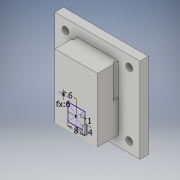
# Autodesk Inventor part: ChipMount
Saved by Autodesk Inventor 2019 (Build 230136000, 136)
## iProperties
Created: 2019-05-13
Part Number: ChipMount
Material: Generic
Document SubType Name: Modeling
Designer: aorfi
Density: 1 g/cm^3
Appearance: Default
Author: aorfi
Autodesk Inventor part; units mm, degrees
ref_plane "YZ Plane" through (0, 0, 0) normal (1, 0, 0) x (0, 1, 0)
ref_plane "XZ Plane" through (0, 0, 0) normal (0, 1, 0) x (-1, 0, 0)
ref_plane "XY Plane" through (0, 0, 0) normal (0, 0, 1) x (1, 0, 0)
sketch "Sketch1" plane through (0, 0, 0) normal (0, 0, 1) x (1, 0, 0)
  line L0 (-20, -20) -> (20, -20)
  line L1 (20, -20) -> (20, 20)
  line L2 (20, 20) -> (-20, 20)
  line L3 (-20, 20) -> (-20, -20)
  line L4 (-20, -20) -> (20, 20) construction
  line L5 (20, -20) -> (-20, 20) construction
  circle A0 centre (0, 0) radius 12.7
  dimension "d0" = 40
  dimension "d51" = 25.4
  constraints: 12 end point, 2 midpoint, 2 parallel, 2 perpendicular, 1 centre point, 1 coincident, 1 horizontal
  measures "d0" distance of L1.end L2.end
  measures "d51" diameter of A0
extrude "Extrusion1" add sketch "Sketch1" along normal mid plane 4 contours L3 L2 L1 L0 | A0
sketch "Sketch2" plane through (0, 0, 2) normal (0, 0, 1) x (1, 0, 0)
  line L0 (-15, 15) -> (15, 15) construction
  line L1 (15, 15) -> (15, -15) construction
  point P0 (0, 0)
  point P1 (0, 15)
  point P2 (-15, -15)
  point P3 (15, 0)
  dimension "d3" = 30
  dimension "d4" = 30
  constraints: 4 end point, 3 vertical alignment, 2 horizontal alignment, 2 midpoint, 1 horizontal, 1 vertical
  measures "d3" distance of L0.start L0.end
  measures "d4" distance of L0.end L1.end
hole "Hole1" at (15, 15, 2) at (-15, 15, 2) at (-15, -15, 2) at (15, -15, 2) direction (0, 0, -1) diameter 3.264 end through all clearance for "Flat Head Machine Screw (82)" size "#4" standard "Ansi Unified Screw Threads"
sketch "Sketch3" plane through (0, 0, 2) normal (0, 0, 1) x (1, 0, 0)
  line L0 (-10, 15) -> (10, 15)
  line L1 (10, 15) -> (10, -15)
  line L2 (10, -15) -> (-10, -15)
  line L3 (-10, -15) -> (-10, 15)
  line L4 (-10, 15) -> (10, -15) construction
  line L5 (10, 15) -> (-10, -15) construction
  point P0 (0, 0)
  dimension "d12" = 20
  dimension "d13" = 30
  constraints: 12 end point, 2 midpoint, 2 parallel, 1 horizontal, 1 perpendicular
  measures "d12" distance of L0.start L0.end
  measures "d13" distance of L0.end L1.end
extrude "Extrusion2" add sketch "Sketch3" along normal blind 10
sketch "Sketch4" plane through (0, 0, 12) normal (0, 0, 1) x (1, 0, 0)
  line L0 (-4, -3.5) -> (4, -3.5)
  line L1 (4, -3.5) -> (4, -11.5)
  line L2 (4, -11.5) -> (-4, -11.5)
  line L3 (-4, -11.5) -> (-4, -3.5)
  line L4 (-4, -3.5) -> (4, -11.5) construction
  line L5 (4, -3.5) -> (-4, -11.5) construction
  line L6 (4, -8.5) -> (5, -8.5)
  line L7 (5, -8.5) -> (5, -12.5)
  line L8 (5, -12.5) -> (1, -12.5)
  line L9 (1, -12.5) -> (1, -11.5)
  line L10 (0, 0) -> (0, -15) construction
  line L11 (10, -15) -> (-10, -15) construction
  point P0 (0, -7.5)
  point P1 (0, -7.5)
  point P2 (0, -7.5)
  point P3 (-6, -1.5)
  dimension "d16" = 8
  dimension "d17" = 1
  dimension "d18" = 4
  dimension "d30" = 6
  dimension "d31" = 6
  constraints: 22 end point, 7 perpendicular, 6 midpoint, 2 horizontal, 2 parallel, 2 point on line, 1 vertical alignment
  measures "d16" distance of L1.end L2.end
  measures "d17" distance of L6.start L6.end
  measures "d18" distance of L6.end L7.end
  measures "d30" horizontal distance of point (0, -7.5) point (-6, -1.5)
  measures "d31" horizontal distance of point (0, -7.5) point (-6, -1.5)
extrude "Extrusion3" add sketch "Sketch4" along normal blind 1 contours L6 L7 L8 L9 L2 L1
hole "Hole3" at (-6, -1.5, 12) direction (0, 0, -1) diameter 1.425 depth 5.692 tip angle 118 thread size "1-64 UNC" class "2B" standard "ANSI Unified Screw Threads"
sketch "Sketch6" plane through (0, 0, 12) normal (0, 0, 1) x (1, 0, 0)
  point P0 (0, 0)
sketch "Sketch7" plane through (0, 0, 12) normal (0, 0, 1) x (1, 0, 0)
  line L0 (0, 0) -> (0, 15) construction
  line L1 (-9, 1) -> (9, 1) construction
  line L2 (9, 1) -> (9, 14) construction
  line L3 (9, 14) -> (-9, 14) construction
  line L4 (-9, 14) -> (-9, 1) construction
  line L5 (-9, 1) -> (9, 14) construction
  line L6 (9, 1) -> (-9, 14) construction
  line L7 (10, 15) -> (-10, 15) construction
  line L8 (9, 4) -> (10, 4)
  line L9 (10, 4) -> (10, 0)
  line L10 (10, 0) -> (6, 0)
  line L11 (6, 0) -> (6, 1)
  line L12 (6, 1) -> (9, 1)
  line L13 (9, 4) -> (9, 1)
  line L14 (-6, 14) -> (-6, 15)
  line L15 (-6, 15) -> (-10, 15)
  line L16 (-10, 15) -> (-10, 11)
  line L17 (-10, 11) -> (-9, 11)
  line L18 (-9, 14) -> (-9, 11)
  line L19 (-9, 14) -> (-6, 14)
  point P0 (0, 7.5)
  dimension "d39" = 18
  dimension "d40" = 1
  dimension "d41" = 4
  dimension "d44" = 13
  constraints: 38 end point, 10 perpendicular, 6 equal length, 4 midpoint, 4 point on line, 3 horizontal, 2 parallel, 2 vertical
  measures "d39" distance of L3.end L2.end
  measures "d40" distance of L8.start L8.end
  measures "d41" distance of L8.end L9.end
  measures "d44" distance of L1.end L2.end
extrude "Extrusion4" [suppressed]
sketch "Sketch8" plane through (-10, 15, 2) normal (0, 1, 0) x (1, 0, 0)
  line L0 (20, 0) -> (20, -10) projected
  line L1 (0, 0) -> (20, 0) projected
  line L2 (10, -10) -> (10, 0) construction
  line L3 (20, -10) -> (0, -10) projected
  arc A0 (20, 0) -> (20, -2.5981) centre (20.75, -1.299) ccw
  line L4 (20, -2.5981) -> (20, 0)
  line L5 (0, 0) -> (0, -10)
  arc A1 (0, -2.5981) -> (0, 0) centre (-0.75, -1.299) ccw
  point P0 (10, 2)
  dimension "d49" = 1.5
  dimension "d50" = 0.75
  constraints: 6 end point, 4 point on circle, 2 centre point, 2 midpoint, 2 point on line, 2 symmetric about line, 1 vertical, 1 other
  measures "d49" radius of A0
  measures "d50" distance from line of L0 A0.centre
extrude "Extrusion5" cut sketch "Sketch8" against normal blind 15 contours L0 A0 | A1 L5
equation "\"d31\" = d30"
body "Solid1"
